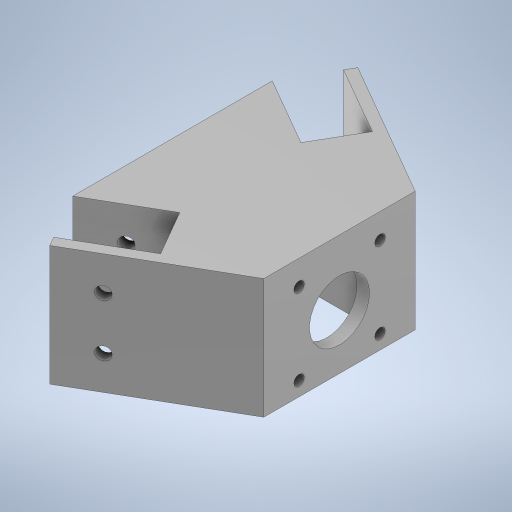
# Autodesk Inventor part: cornerBracket
Saved by Autodesk Inventor 2024.2 (Build 282272000, 272)
## iProperties
Created: 2024-03-31
Part Number: cornerBracket
Material: ABS Plastic
Document SubType Name: Modeling
Designer: Robin
Density: 1.06 g/cm^3
Appearance: Smooth - White
Author: Robin
Autodesk Inventor part; units mm, degrees
ref_plane "YZ Plane" through (0, 0, 0) normal (1, 0, 0) x (0, 1, 0)
ref_plane "XZ Plane" through (0, 0, 0) normal (0, 1, 0) x (-1, 0, 0)
ref_plane "XY Plane" through (0, 0, 0) normal (0, 0, 1) x (1, 0, 0)
sketch "Sketch1" plane through (0, 0, 0) normal (0, 1, 0) x (-1, 0, 0)
  line L0 (114.191, 65.9282) -> (0, 0)
  line L1 (0, 0) -> (114.191, -65.9282)
  line L2 (114.191, -65.9282) -> (114.191, 65.9282)
  line L3 (-22.8382, 0) -> (137.0292, 0) projected
  line L4 (55, 21.5) -> (55, -21.5)
  line L5 (55, 21.5) -> (114.191, 21.5)
  line L6 (114.191, 21.5) -> (114.191, -21.5)
  line L7 (114.191, -21.5) -> (55, -21.5)
  line L8 (50.2295, 29) -> (50.2295, -29)
  line L9 (114.191, -61.3094) -> (78.2102, -40.5359)
  line L10 (78.2102, -40.5359) -> (88.2102, -23.2154)
  line L11 (88.2102, -23.2154) -> (114.191, -38.2154)
  line L12 (114.191, 38.2154) -> (88.2102, 23.2154)
  line L13 (88.2102, 23.2154) -> (78.2102, 40.5359)
  line L14 (78.2102, 40.5359) -> (114.191, 61.3094)
  line L15 (114.191, -38.2154) -> (102.191, -59)
  line L16 (114.191, 38.2154) -> (102.191, 59)
  point P0 (55, 0)
  point P1 (114.191, -21.5)
  point P2 (114.191, 21.5)
  dimension "d1" = 60
  dimension "d3" = 150
  dimension "d4" = 43
  dimension "d6" = 55
  dimension "d8" = 20
  dimension "d9" = 20
  dimension "d10" = 4
  dimension "d11" = 4
  dimension "d54" = 58
  dimension "d55" = 60
  dimension "d56" = 30
  dimension "d57" = 30
  constraints: 32 end point, 9 perpendicular, 8 point on line, 4 parallel, 1 collinear, 1 horizontal, 1 horizontal alignment, 1 midpoint
  measures "d1" angle of L1 L0
  measures "d3" angle of L3 L1
  measures "d4" distance of L4.start L4.end
  measures "d6" distance from line of L0.end L4
  measures "d8" distance between parallel lines of L12 L14
  measures "d9" distance between parallel lines of L11 L9
  measures "d10" distance between parallel lines of L0 L14
  measures "d11" distance between parallel lines of L1 L9
  measures "d54" distance of L8.start L8.end
  measures "d55" distance of L8.end L15.end
  measures "d56" distance of L10.end L11.end
  measures "d57" distance of L12.start L12.end
extrude "Extrusion1" add sketch "Sketch1" along normal blind 46 contours L2 L14 L16 L0 | L16 L14 L13 L12 L2 L5 L4 L3 L8 L0 | L3 L4 L7 L2 L11 L10 L9 L15 L1 L8 | L15 L9 L2 L1
sketch "Sketch2" plane through (0, 46, 0) normal (0, 1, 0) x (1, 0, 0)
  line L0 (-114.191, -21.5) -> (-114.191, -38.2154) projected
  line L1 (-114.191, 21.5) -> (-55, 21.5) projected
  line L2 (-114.191, -21.5) -> (-55, -21.5)
  line L3 (-55, -21.5) -> (-55, 21.5)
  line L4 (-55, 21.5) -> (-114.191, 21.5)
  line L5 (-114.191, 21.5) -> (-114.191, -21.5)
  point P0 (0, 0)
  point P1 (-114.191, 21.5)
  constraints: 8 end point, 2 parallel, 1 horizontal, 1 perpendicular
extrude "Extrusion2" add sketch "Sketch2" against normal blind 4
sketch "Sketch3" plane through (-55, 0, -21.5) normal (-1, 0, 0) x (0, 0, 1)
  circle A0 centre (21.5, 21) radius 11.5
  line L0 (0, 0) -> (43, 0) projected
  circle A1 centre (6, 5.5) radius 2
  circle A2 centre (37, 5.5) radius 2
  circle A3 centre (37, 36.5) radius 2
  circle A4 centre (6, 36.5) radius 2
  line L1 (0, 0) -> (0, 42) projected
  line L2 (37, 5.5) -> (6, 36.5)
  line L3 (6, 36.5) -> (6, 5.5)
  line L4 (6, 5.5) -> (37, 36.5)
  point P0 (21.5, 0)
  point P1 (21.5, 0)
  dimension "d18" = 21
  dimension "d19" = 23
  dimension "d20" = 31
  dimension "d21" = 31
  dimension "d22" = 4
  dimension "d23" = 4
  dimension "d24" = 4
  dimension "d25" = 4
  constraints: 6 end point, 5 centre point, 3 midpoint, 3 vertical alignment, 2 horizontal alignment, 1 vertical
  measures "d18" distance from line of L0 A0.centre
  measures "d19" diameter of A0
  measures "d20" distance of L3.end L2.start
  measures "d21" distance of L3.end L2.end
  measures "d22" diameter of A1
  measures "d23" diameter of A2
  measures "d24" diameter of A3
  measures "d25" diameter of A4
extrude "Extrusion3" cut sketch "Sketch3" against normal blind 46 contours A0 L2 L4 | L4 L2 A0 | A0 L4 L2 | L2 L4 A0 | L2 L3 A4 | A4 L3 L2 | L4 L3 A1 | A1 L3 L4 | A2 | A3
sketch "Sketch4" plane through (0, 0, 0) normal (0, -1, 0) x (1, 0, 0)
  line L0 (-114.191, -38.2154) -> (-114.191, 38.2154) projected
  line L1 (-114.191, -38.2154) -> (-102.191, -59)
  line L2 (-50.2295, -29) -> (-114.191, -65.9282) projected
  line L3 (-114.191, -65.9282) -> (-114.191, -38.2154)
  line L4 (-114.191, 38.2154) -> (-102.191, 59)
  line L5 (-114.191, 65.9282) -> (-50.2295, 29) projected
  line L6 (-114.191, 65.9282) -> (-114.191, 38.2154)
  line L7 (-102.191, 59) -> (-114.191, 65.9282)
  line L8 (-102.191, -59) -> (-114.191, -65.9282)
  line L9 (-102.191, 59) -> (-114.684, 66.2128)
  line L10 (-102.191, 59) -> (-114.191, 38.2154)
  point P0 (0, 0)
  constraints: 16 end point, 4 point on line, 2 collinear, 2 perpendicular, 2 vertical alignment, 1 vertical
extrude "Extrusion4" cut sketch "Sketch4" against normal through all
sketch "Sketch5" plane through (-50.2295, 0, 29) normal (0.5, 0, 0.8660254) x (0.8660254, 0, -0.5)
  circle A0 centre (-45, 13) radius 2.5
  circle A1 centre (-45, 33) radius 2.5
  line L0 (-60, 46) -> (-60, 0) projected
  line L1 (-60, 0) -> (0, 0) projected
  point P0 (58, 0)
  dimension "d34" = 20
  dimension "d35" = 15
  dimension "d36" = 13
  dimension "d37" = 5
  dimension "d38" = 5
  constraints: 2 centre point, 1 vertical alignment
  measures "d34" distance of A1.centre A0.centre
  measures "d35" distance from line of L0 A0.centre
  measures "d36" distance from line of L1 A0.centre
  measures "d37" diameter of A0
  measures "d38" diameter of A1
extrude "Extrusion5" cut sketch "Sketch5" against normal through all
sketch "Sketch6" plane through (-50.2295, 0, -29) normal (0.5, 0, -0.8660254) x (-0.8660254, 0, -0.5)
  circle A0 centre (45, 10) radius 2.5
  circle A1 centre (45, 30) radius 2.5
  line L0 (0, 0) -> (60, 0) projected
  line L1 (60, 0) -> (60, 46) projected
  point P0 (-58, 0)
  dimension "d41" = 20
  dimension "d42" = 10
  dimension "d43" = 15
  dimension "d44" = 5
  dimension "d45" = 5
  constraints: 2 centre point, 1 vertical alignment
  measures "d41" distance of A1.centre A0.centre
  measures "d42" distance from line of L0 A0.centre
  measures "d43" distance from line of L1 A0.centre
  measures "d44" diameter of A1
  measures "d45" diameter of A0
extrude "Extrusion6" cut sketch "Sketch6" against normal through all
sketch "Sketch7" plane through (0, 0, 0) normal (0, -1, 0) x (1, 0, 0)
  line L0 (-114.191, 21.5) -> (-55, 21.5) projected
  line L1 (-95.2391, 21.5) -> (-114.191, 32.4419)
  line L2 (-114.191, -38.2154) -> (-114.191, 38.2154) projected
  line L3 (-114.191, 21.5) -> (-95.2391, 21.5)
  line L4 (-114.191, 21.5) -> (-114.191, 32.4419)
  line L5 (-114.191, 38.2154) -> (-88.2102, 23.2154) projected
  point P0 (0, 0)
  dimension "d48" = 5
  constraints: 6 end point, 2 point on line, 1 horizontal, 1 parallel, 1 perpendicular
  measures "d48" distance between parallel lines of L5 L1
sketch "Sketch8" plane through (0, 0, 0) normal (0, -1, 0) x (1, 0, 0)
  line L0 (-55, -21.5) -> (-114.191, -21.5) projected
  line L1 (-95.2391, -21.5) -> (-114.191, -32.4419)
  line L2 (-114.191, -38.2154) -> (-114.191, -21.5) projected
  line L3 (-114.191, -21.5) -> (-95.2391, -21.5)
  line L4 (-114.191, -32.4419) -> (-114.191, -21.5)
  line L5 (-88.2102, -23.2154) -> (-114.191, -38.2154) projected
  point P0 (0, 0)
  dimension "d49" = 5
  constraints: 6 end point, 2 point on line, 1 horizontal, 1 parallel, 1 perpendicular
  measures "d49" distance between parallel lines of L5 L1
extrude "Extrusion7" cut sketch "Sketch8" against normal up to surface (42 mm away)
extrude "Extrusion8" cut sketch "Sketch7" against normal up to surface (42 mm away)
body "Solid1"
